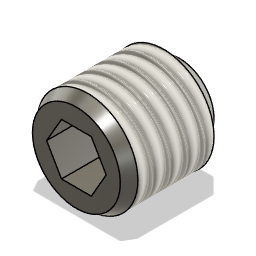
blind control (Autodesk Fusion 360 archive; units mm, degrees)
design "Hexagon Socket Set Screw ISO 4026 - M3 x 3 Steel 4.6 Plain"
description: Hexagon Socket Set Screw ISO 4026 - M3 x 3
Autodesk Fusion 360 part; units mm, degrees
sketch "Sketch9" plane through (0, 0, 0) normal (0, 1, 0) x (1, 0, 0)
  line L0 (0, 0) -> (-1.5, 0)
  line L1 (-1.5, 0) -> (-1.5, 3)
  line L2 (-1.5, 3) -> (0, 3)
  line L3 (0, 3) -> (0, 0)
  dimension "d143" = 3
  dimension "d144" = 3
  constraint coincident L0.start L3.end
  constraint horizontal L0
  constraint perpendicular L0 L1
  constraint perpendicular L1 L2
  constraint perpendicular L0 L3
  measures "d144" distance of L0.end L1.end
revolve "Revolve4" add sketch "Sketch9" angle 360 about axis through (0, 0, -3) along (0, 0, 1)
sketch "Sketch7" plane through (0, 0, 0) normal (0, 0, 1) x (1, 0, 0)
  line L0 (-1.5, 0) -> (1.5, 0)
  line L1 (0, 0) -> (-0.866, 0)
  line L2 (-0.433, 0.75) -> (-0.866, 0)
  line L3 (0, 0) -> (-0.433, 0.75)
  circle A0 centre (0, 0) radius 1.5
  dimension "d120" = 60
  dimension "d121" = 60
  dimension "d122" = 0.75
  constraint horizontal L0
  constraint coincident L1.start L0
  constraint coincident L0 L1.end
  constraint coincident L0.end A0
  constraint coincident L0.start A0
  constraint coincident L1.start L3.start
  measures "d120" angle of L1 L3
  measures "d121" angle of L2 L3
  measures "d122" distance of L1.start L2
extrude "Extrude6" cut sketch "Sketch7" against normal blind 1.2 contours L0 L1 L2 L3
pattern_circular "C-Pattern1" count 6 over 360 about axis through (0, 0, 1.75) along (0, 0, 1) of "Extrude6"
extrude "Extrude7" cut 1 faces at (-0.1443, 0.25, -1.2) along direction (0, 0, -1) blind 1.2 draft -60
thread "Thread3" "ISO Metric profile 3.0 M3x0.5 6g" major diameter 2.927 minor diameter 2.3555 pitch 0.5 angle 60 resizes the face on face at (-1.4981, 0.0748, -1)
sketch "Sketch8" plane through (0, 0, 0) normal (0, 1, 0) x (1, 0, 0)
  line L0 (-1.53, 3) -> (-1.53, 2.47)
  line L1 (-1.53, 2.47) -> (-1, 3)
  line L2 (-1.53, 3) -> (0, 3)
  line L3 (0, 0) -> (-1.53, 0)
  line L4 (-1.53, 0) -> (-1.53, 0.4391)
  line L5 (-1.53, 0.4391) -> (-1.2765, 0)
  line L6 (0, 3) -> (0, 0)
  point P0 (0, 3)
  dimension "d134" = 45
  dimension "d136" = 0.2535
  dimension "d137" = 1.53
  dimension "d138" = 60
  dimension "d153" = 1.53
  dimension "d154" = 1
  constraint vertical L0
  constraint coincident L1.end L2
  constraint perpendicular L3 L4
  constraint coincident L3 L5.end
  constraint coincident L3.start L6.end
  constraint perpendicular L3 L6
  constraint perpendicular L2 L6
  constraint coincident P0 L2.end
  measures "d134" angle of L0 L1
  measures "d136" distance of L3.end L5.end
  measures "d137" distance of L3.start L3.end
  measures "d138" angle of L3 L5
  measures "d153" horizontal distance of L0.start L3.start
  measures "d154" horizontal distance of L1.end L3.start
revolve "Revolve5" cut sketch "Sketch8" angle 360 about axis through (0, 0, 1.75) along (0, 0, 1)
equation "adsk_nomlen = 3.00 mm"
equation "adsk_nomdia = 3.00 mm"
equation "adsk_phildepth = 1.20 mm"
equation "adsk_endpointwidth = 2.00 mm"
equation "adsk_chamang = 60.00 deg"
equation "d122 = adsk_philwidth / 2"
equation "adsk_philwidth = 1.50 mm"
equation "d134 = adsk_endpointang"
equation "d136 = ( adsk_nomdia - adsk_philwidth * 1.155 ) / 5"
equation "d137 = adsk_nomdia * 0.51"
equation "d138 = adsk_chamang"
equation "adsk_endpointang = 45.00 deg"
equation "d143 = adsk_nomdia"
equation "d144 = adsk_nomlen"
equation "d146 = -adsk_phildepth"
equation "d148 = -adsk_phildepth"
equation "d153 = adsk_nomdia * 0.51"
equation "d154 = adsk_endpointwidth / 2"

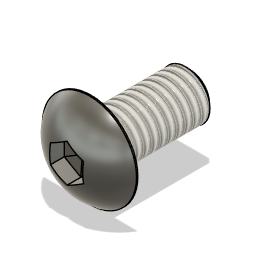
design "Button Head Screw JIS B 1174 - M3 x 6 Steel 4.6 Plain"
description: Button Head Screw JIS B 1174 - M3 x 6
Autodesk Fusion 360 part; units mm, degrees
sketch "Sketch1" plane through (0, 0, 0) normal (0, 1, 0) x (1, 0, 0)
  line L0 (-1.5, 0) -> (-1.5, 6)
  line L1 (-1.5, 6) -> (0, 6)
  line L2 (0, 6) -> (0, -1.65)
  line L3 (-1.5, 0) -> (-2.85, 0)
  line L4 (-2.85, 0) -> (-2.85, -0.0825)
  arc A0 (-2.85, -0.0825) -> (0, -1.65) centre (0, 1.7247) ccw
  dimension "d9" = 3
  dimension "d66" = 5.7
  dimension "d68" = 6
  dimension "d78" = 1.65
  dimension "d79" = 0.0825
  constraint perpendicular L0 L1
  constraint collinear origin L2.end L1.end
  constraint perpendicular L0 L3
  constraint coincident origin L3
  constraint vertical L0
  constraint vertical L2
  constraint vertical L4
  constraint coincident L2 A0.centre
  constraint coincident L2.end A0.end
  measures "d68" distance of origin L1.end
  measures "d78" vertical distance of L2.end L3.end
  measures "d79" distance of L3.end L4.end
revolve "Revolve1" add sketch "Sketch1" angle 360 about axis through (0, 0, -6) along (0, 0, 1)
ref_plane "WorkPlane1" through (0, 0, 1.65) normal (0, 0, 1) x (1, 0, 0)
sketch "Sketch6" plane through (0, 0, 1.65) normal (0, 0, 1) x (1, 0, 0)
  line L0 (-1, 0) -> (1, 0) construction
  line L1 (0, 0) -> (-1, 0.5774)
  line L2 (-1, -0.5774) -> (-1, 0.5774)
  line L3 (-1, -0.5774) -> (0, 0)
  dimension "d72" = 2
  dimension "d91" = 150
  constraint horizontal L0
  constraint midpoint L1.start L0
  constraint coincident L1.start L3.end
  constraint perpendicular L0 L2
  constraint midpoint L0.start L2
  constraint coincident L1.end L2.end
  measures "d72" distance of L0.start L0.end
  measures "d91" angle of L0 L1
extrude "Extrude1" cut sketch "Sketch6" against normal blind 1.04
pattern_circular "C-Pattern1" count 6 over 360 about axis through (0, 0, 1.75) along (0, 0, 1) of "Extrude1"
extrude "Extrude2" cut 1 faces at (0, 0, 0.61) along direction (0, 0, -1) blind 1.04 draft -85
thread "Thread2" "ISO Metric profile 3.0 M3x0.5 6g" major diameter 2.927 minor diameter 2.3555 pitch 0.5 angle 60 resizes the face on face at (-1.4925, 0.1494, -4) from (0, 0, -1) to (0, 0, -6)
sketch "Sketch5" plane through (0, 0, 0) normal (0, 1, 0) x (1, 0, 0)
  line L0 (0, 6) -> (0, -1.65)
  line L1 (0, 6) -> (-1.53, 6)
  line L2 (-1.53, 6) -> (-1.53, 5.6933)
  line L3 (-1.53, 5.6933) -> (-1.1933, 6)
  dimension "d92" = 1.1933
  dimension "d93" = 1.53
  dimension "d94" = 0.3067
  constraint coincident L0.start L1.start
  constraint perpendicular L0 L1
  constraint perpendicular L1 L2
  constraint coincident L1 L3.end
  measures "d92" horizontal distance of origin L3.end
  measures "d93" horizontal distance of origin L1.end
  measures "d94" distance of L1.end L2.end
revolve "Revolve2" cut sketch "Sketch5" angle 360 about axis through (0, 0, -6) along (0, 0, 1)
equation "d9 = adsk_nomdia"
equation "adsk_nomlen = 6.00 mm"
equation "adsk_headh = 1.65 mm"
equation "adsk_headdia = 5.70 mm"
equation "adsk_nomdia = 3.00 mm"
equation "adsk_waflat = 2.00 mm"
equation "d31 = -adsk_keyend"
equation "adsk_keyend = 1.04 mm"
equation "d66 = adsk_headdia"
equation "d68 = adsk_nomlen"
equation "d71 = adsk_headh"
equation "d72 = adsk_waflat"
equation "d76 = -adsk_keyend"
equation "d78 = adsk_headh"
equation "d79 = adsk_headh * 0.05"
equation "adsk_thrlen = 5.00 mm"
equation "adsk_endpointdia = 2.38655 mm"
equation "adsk_startlen = 0.306725 mm"
equation "d92 = adsk_endpointdia / 2"
equation "d93 = adsk_nomdia * 0.51"
equation "d94 = adsk_startlen"
equation "d96 = adsk_thrlen"

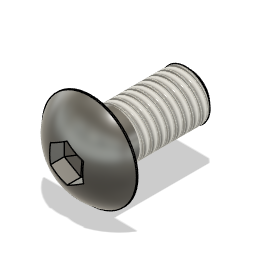
design "Hexagon Socket Button Head Screw ISO 7380-1 - M3 x 6 Steel 4.6 Plain"
description: Hexagon Socket Button Head Screw ISO 7380-1 - M3 x 6
Autodesk Fusion 360 part; units mm, degrees
sketch "Sketch1" plane through (0, 0, 0) normal (0, 1, 0) x (1, 0, 0)
  line L0 (-1.5, 0) -> (-1.5, 6)
  line L1 (-1.5, 6) -> (0, 6)
  line L2 (0, 6) -> (0, -1.65)
  line L3 (-1.5, 0) -> (-2.85, 0)
  line L4 (-2.85, 0) -> (-2.85, -0.0825)
  arc A0 (-2.85, -0.0825) -> (0, -1.65) centre (0, 1.7247) ccw
  dimension "d9" = 3
  dimension "d66" = 5.7
  dimension "d68" = 6
  dimension "d78" = 1.65
  dimension "d79" = 0.0825
  constraint perpendicular L0 L1
  constraint collinear origin L2.end L1.end
  constraint perpendicular L0 L3
  constraint coincident origin L3
  constraint vertical L0
  constraint vertical L2
  constraint vertical L4
  constraint coincident L2 A0.centre
  constraint coincident L2.end A0.end
  measures "d68" distance of origin L1.end
  measures "d78" vertical distance of L2.end L3.end
  measures "d79" distance of L3.end L4.end
revolve "Revolve1" add sketch "Sketch1" angle 360 about axis through (0, 0, -6) along (0, 0, 1)
ref_plane "WorkPlane1" through (0, 0, 1.65) normal (0, 0, 1) x (1, 0, 0)
sketch "Sketch6" plane through (0, 0, 1.65) normal (0, 0, 1) x (1, 0, 0)
  line L0 (-1, 0) -> (1, 0) construction
  line L1 (0, 0) -> (-1, 0.5774)
  line L2 (-1, -0.5774) -> (-1, 0.5774)
  line L3 (-1, -0.5774) -> (0, 0)
  dimension "d72" = 2
  dimension "d91" = 150
  constraint horizontal L0
  constraint midpoint L1.start L0
  constraint coincident L1.start L3.end
  constraint perpendicular L0 L2
  constraint midpoint L0.start L2
  constraint coincident L1.end L2.end
  measures "d72" distance of L0.start L0.end
  measures "d91" angle of L0 L1
extrude "Extrude1" cut sketch "Sketch6" against normal blind 1.04
pattern_circular "C-Pattern1" count 6 over 360 about axis through (0, 0, 1.75) along (0, 0, 1) of "Extrude1"
extrude "Extrude2" cut 1 faces at (0, 0, 0.61) along direction (0, 0, -1) blind 1.04 draft -85
thread "Thread2" "ISO Metric profile 3.0 M3x0.5 6g" major diameter 2.927 minor diameter 2.3555 pitch 0.5 angle 60 resizes the face on face at (-1.4925, 0.1494, -4) from (0, 0, -1.5) to (0, 0, -6)
sketch "Sketch5" plane through (0, 0, 0) normal (0, 1, 0) x (1, 0, 0)
  line L0 (0, 6) -> (0, -1.65)
  line L1 (0, 6) -> (-1.53, 6)
  line L2 (-1.53, 6) -> (-1.53, 5.7)
  line L3 (-1.53, 5.7) -> (-1.2, 6)
  dimension "d92" = 1.2
  dimension "d93" = 1.53
  dimension "d94" = 0.3
  constraint coincident L0.start L1.start
  constraint perpendicular L0 L1
  constraint perpendicular L1 L2
  constraint coincident L1 L3.end
  measures "d92" horizontal distance of origin L3.end
  measures "d93" horizontal distance of origin L1.end
  measures "d94" distance of L1.end L2.end
revolve "Revolve2" cut sketch "Sketch5" angle 360 about axis through (0, 0, -6) along (0, 0, 1)
equation "d9 = adsk_nomdia"
equation "adsk_nomlen = 6.00 mm"
equation "adsk_headh = 1.65 mm"
equation "adsk_headdia = 5.70 mm"
equation "adsk_nomdia = 3.00 mm"
equation "adsk_waflat = 2.00 mm"
equation "d31 = -adsk_keyend"
equation "adsk_keyend = 1.04 mm"
equation "d66 = adsk_headdia"
equation "d68 = adsk_nomlen"
equation "d71 = adsk_headh"
equation "d72 = adsk_waflat"
equation "d76 = -adsk_keyend"
equation "d78 = adsk_headh"
equation "d79 = adsk_headh * 0.05"
equation "adsk_thrlen = 4.50 mm"
equation "adsk_endpointdia = adsk_nomdia - 2 * adsk_startlen"
equation "adsk_startlen = 0.1 * adsk_nomdia"
equation "d92 = adsk_endpointdia / 2"
equation "d93 = adsk_nomdia * 0.51"
equation "d94 = adsk_startlen"
equation "d96 = adsk_thrlen"
